Base Motor Brackey_v3 (Autodesk Fusion 360 design; units mm, degrees)
Autodesk Fusion 360 part; units mm, degrees
sketch "Sketch1" plane through (0, 0, 0) normal (0, 0, 1) x (1, 0, 0)
  line L0 (0, 0) -> (-30.23, 0) construction
  line L1 (-30.23, 0) -> (-30.23, 30) construction
  line L2 (-30.23, 30) -> (-37.23, 30)
  line L3 (-37.23, 30) -> (-37.23, -40)
  line L4 (-37.23, -40) -> (-30.23, -40)
  line L5 (-30.23, 0) -> (-30.23, 30)
  line L6 (-30.23, 0) -> (0, 0)
  line L7 (0, 0) -> (0, -40)
  line L8 (0, -40) -> (-30.23, -40)
  line L9 (0, 0) -> (0, -40)
  line L10 (0, -40) -> (30.23, -40)
  line L11 (37.23, -40) -> (30.23, -40)
  line L12 (37.23, 30) -> (37.23, -40)
  line L13 (30.23, 30) -> (37.23, 30)
  line L14 (30.23, 0) -> (30.23, 30)
  line L15 (0, 0) -> (30.23, 0)
  dimension "d1" = 30.23
  dimension "d2" = 30
  dimension "d3" = 7
  dimension "d4" = 70
  dimension "d5" = 30.23
  dimension "d6" = 40
  constraint horizontal L0
  constraint vertical L1
  constraint coincident L0.start L6.end
  constraint horizontal L2
  constraint vertical L3
  constraint horizontal L4
  constraint vertical L5
  constraint horizontal L6
  constraint vertical L7
  constraint horizontal L8
  constraint symmetric L0.start L7 L6.end
  constraint symmetric L0.end L7 L14.start
  constraint symmetric L1.end L7 L13.start
  constraint symmetric L2.end L7 L12.start
  constraint symmetric L3.end L7 L11.start
  constraint symmetric L4.end L7 L10.end
  constraint symmetric L8.start L7 L9.end
  measures "d1" distance of L0.start L0.end
  measures "d2" distance of L0.end L1.end
  measures "d3" distance of L1.end L2.end
  measures "d4" distance of L1.end L4.end
  measures "d5" distance of L0.end L0.start
  measures "d6" distance of L0.end L4.end
extrude "Extrude1" add sketch "Sketch1" along normal blind 15
hole "Hole1" at (37.23, 20, 7.5) direction (-1, 0, 0) diameter 4 end through all
sketch "Sketch2" plane through (0, 0, 15) normal (0, 0, 1) x (-1, 0, 0)
  line L0 (30.23, 0) -> (30.23, -30)
  line L1 (30.23, -30) -> (37.23, -30)
  line L2 (37.23, -30) -> (37.23, 40)
  line L3 (37.23, 40) -> (-37.23, 40)
  line L4 (-37.23, 40) -> (-37.23, -30)
  line L5 (-37.23, -30) -> (-30.23, -30)
  line L6 (-30.23, -30) -> (-30.23, 0)
  line L7 (-30.23, 0) -> (30.23, 0)
  line L8 (0, 0) -> (0, -15.4) construction
  line L9 (37.23, 24.6) -> (-37.23, 24.6)
  line L10 (-37.23, 24.6) -> (-37.23, 40)
  line L11 (-37.23, 40) -> (37.23, 40)
  line L12 (37.23, 40) -> (37.23, 24.6)
  dimension "d14" = 15.4
  dimension "d16" = 40
  constraint coincident L8.start origin
  constraint perpendicular L7 L8
  constraint horizontal L9
  constraint vertical L10
  constraint horizontal L11
  constraint vertical L12
  constraint coincident L3.end L4.start
  constraint coincident L2 L9.start
  measures "d14" distance of L8.start L8.end
  measures "d16" distance of L8.end L9
extrude "Extrude2" add sketch "Sketch2" along normal blind 49.5 contours L2 L3 L4 L9 L10 L11 L12
sketch "Sketch3" plane through (0, 0, 64.5) normal (0, 0, 1) x (-1, 0, 0)
  line L0 (37.23, 40) -> (-37.23, 40)
  line L1 (-37.23, 40) -> (-37.23, 24.6)
  line L2 (-37.23, 24.6) -> (37.23, 24.6)
  line L3 (37.23, 24.6) -> (37.23, 40)
  spline S0 degree 2 poles (37.23, 24.6) (0, -58.216) (-37.23, 24.6) knots 0 0 0 14.204514 14.204514 14.204514 weights 1 2.708153 1
  line L4 (37.23, 24.6) -> (37.23, 40)
  line L5 (-37.23, 40) -> (-37.23, 24.6)
  line L6 (-30.23, 0, -49.5) -> (30.23, 0, -49.5) construction
  line L7 (0, 24.6) -> (0, -15.4) construction
  circle A0 centre (0, -15.4) radius 12.75 construction
  circle A1 centre (0, -2.65) radius 1.5
  circle A2 centre (-12.75, -15.4) radius 1.5
  circle A3 centre (0, -28.15) radius 1.5
  circle A4 centre (12.75, -15.4) radius 1.5
  circle A5 centre (0, -15.4) radius 6.5
  dimension "d21" = 40
  dimension "d22" = 25.5
  dimension "d23" = 3
  dimension "d25" = 360
  dimension "d28" = 13
  constraint coincident L1.end L2.start
  constraint coincident L2.end L3.start
  constraint coincident L0.start L3.end
  constraint coincident L0.end L1.start
  constraint midpoint L2 L7.start
  constraint perpendicular L2 L7
  constraint coincident L7.end A0.centre
  constraint coincident A0 A1.centre
  constraint coincident L7 A1.centre
  constraint concentric A0 A5
  measures "d21" distance of L7.start L7.end
  measures "d22" diameter of A0
  measures "d23" diameter of A1
  measures "d28" diameter of A5
extrude "Extrude3" add sketch "Sketch3" along normal blind 5
sketch "Sketch4" plane through (0, 0, 69.5) normal (0, 0, 1) x (-1, 0, 0)
  circle A0 centre (12.75, -15.4) radius 1.5
  circle A1 centre (0, -28.15) radius 1.5
  circle A2 centre (0, -2.65) radius 1.5
  circle A3 centre (-12.75, -15.4) radius 1.5
  circle A4 centre (0, -15.4) radius 6.5
  line L0 (37.23, 24.6) -> (37.23, 40)
  line L1 (37.23, 40) -> (-37.23, 40)
  line L2 (-37.23, 40) -> (-37.23, 24.6)
  spline S0 degree 2 poles (-37.23, 24.6) (0, -58.216) (37.23, 24.6) knots -14.204514 -14.204514 -14.204514 0 0 0 weights 1 2.708153 1
  line L3 (9, -9.9) -> (-9, -9.9) construction
  line L4 (-9, -9.9) -> (-9, -20.9) construction
  line L5 (-9, -20.9) -> (9, -20.9) construction
  line L6 (9, -20.9) -> (9, -9.9) construction
  line L7 (9, -9.9) -> (-9, -20.9) construction
  line L8 (-9, -9.9) -> (9, -20.9) construction
  circle A5 centre (9, -20.9) radius 1
  circle A6 centre (-9, -20.9) radius 1
  circle A7 centre (9, -9.9) radius 1
  circle A8 centre (-9, -9.9) radius 1
  point P0 (0, -15.4)
  dimension "d29" = 18
  dimension "d30" = 11
  dimension "d31" = 2
  dimension "d32" = 2
  dimension "d33" = 2
  dimension "d34" = 2
  constraint horizontal L3
  constraint perpendicular L3 L4
  constraint parallel L3 L5
  constraint parallel L4 L6
  constraint coincident L7 P0
  constraint coincident L8 P0
  constraint coincident P0 A4.centre
  constraint coincident L5.end L6.start
  constraint coincident L4.end L5.start
  constraint coincident L3.start L6.end
  constraint coincident L3.end L4.start
  measures "d29" distance of L4.end L5.end
  measures "d30" distance of L3.end L4.end
  measures "d31" diameter of A5
  measures "d32" diameter of A6
  measures "d33" diameter of A7
  measures "d34" diameter of A8
extrude "Extrude4" cut sketch "Sketch4" against normal blind 7 contours A5 | A6 | A7 | A8
sketch "Sketch5" plane through (0, 0, 69.5) normal (0, 0, 1) x (-1, 0, 0)
  circle A0 centre (-9, -20.9) radius 1
  circle A1 centre (-9, -9.9) radius 1
  circle A2 centre (9, -20.9) radius 1
  circle A3 centre (9, -9.9) radius 1
  circle A4 centre (12.75, -15.4) radius 1.5
  circle A5 centre (0, -28.15) radius 1.5
  circle A6 centre (0, -2.65) radius 1.5
  circle A7 centre (-12.75, -15.4) radius 1.5
  circle A8 centre (0, -15.4) radius 6.5
  line L0 (37.23, 24.6) -> (37.23, 40)
  line L1 (37.23, 40) -> (-37.23, 40)
  line L2 (-37.23, 40) -> (-37.23, 24.6)
  spline S0 degree 2 poles (-37.23, 24.6) (0, -58.216) (37.23, 24.6) knots -14.204514 -14.204514 -14.204514 0 0 0 weights 1 2.708153 1
  circle A9 centre (12.75, -15.4) radius 2.5
  circle A10 centre (0, -2.65) radius 2.5
  circle A11 centre (-12.75, -15.4) radius 2.5
  circle A12 centre (0, -28.15) radius 2.5
  dimension "d37" = 5
  dimension "d39" = 360
  constraint concentric A4 A9
  measures "d37" diameter of A9
extrude "Extrude5" cut sketch "Sketch5" against normal blind 3 contours A9 | A10 | A11 | A12
extrude "Extrude6" cut 1 faces at (-10.0767, 0, 10) along direction (0, -1, 0) blind 5
fillet "Fillet1" radius 4 1 edges at (0, -40, 69.5)
fillet "Fillet2" radius 3.5 2 edges at (-30.23, 30, 7.5) (30.23, 30, 7.5)
equation "d1 = ( 60.46 / 2 ) * 1 mm"
